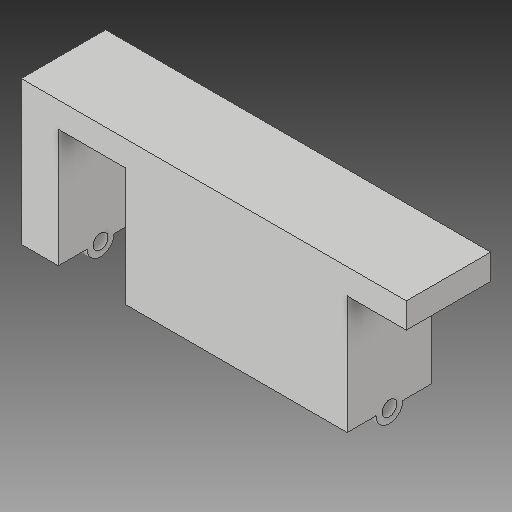
# Autodesk Inventor part: Arm_Base
Saved by Autodesk Inventor 2017 (Build 210142000, 142)
## iProperties
Created: 2016-12-31
Part Number: Arm_Base
Material: Generic
Document SubType Name: Modeling
Designer: Samanth
Density: 1 g/cm^3
Appearance: Default
Author: Samanth
Autodesk Inventor part; units mm, degrees
ref_plane "YZ Plane" through (0, 0, 0) normal (1, 0, 0) x (0, 1, 0)
ref_plane "XZ Plane" through (0, 0, 0) normal (0, 1, 0) x (-1, 0, 0)
ref_plane "XY Plane" through (0, 0, 0) normal (0, 0, 1) x (1, 0, 0)
sketch "Sketch1" plane through (0, 0, 0) normal (0, 0, 1) x (1, 0, 0)
  line L0 (0, 0) -> (55, 0)
  line L1 (0, 0) -> (-76, 0)
  line L2 (-116, 0) -> (-138, 0)
  line L3 (-138, 0) -> (-138, 70)
  line L4 (-138, 70) -> (-138, 85)
  line L5 (-138, 85) -> (-116, 85)
  line L6 (-116, 0) -> (-116, 70)
  line L7 (-116, 70) -> (-76, 70)
  line L8 (-76, 70) -> (-76, 0)
  line L9 (90, 70) -> (90, 85)
  line L10 (90, 85) -> (-116, 85)
  line L11 (55, 0) -> (55, 70)
  line L12 (55, 70) -> (90, 70)
  line L13 (55, 0) -> (-76, 0)
  line L14 (-116, 0) -> (-117.6, 0)
  line L15 (-117.6, 0) -> (-117.6, 71.4164)
  line L16 (-117.6, 71.4164) -> (-74.4045, 71.4164)
  line L17 (-74.4045, 71.4164) -> (-74.4045, 0)
  line L18 (-138, 0) -> (-152.8138, 0)
  line L19 (-152.8138, 0) -> (-152.8138, 85)
  line L20 (-152.8138, 85) -> (-138, 85)
  dimension "d20" = 1.6
  constraints: 42 end point, 10 perpendicular, 4 point on line, 4 vertical, 2 horizontal, 1 collinear
  measures "d20" distance of L2.start L14.end
extrude "Extrusion1" add sketch "Sketch1" along normal blind 50 contours L1 L17 L16 L15 L2 L3 L4 L5 L10 L9 L12 L11 L0 | L1 L8 L7 L6 L2 L15 L16 L17
sketch "Sketch2" plane through (0, 0, 0) normal (1, 0, 0) x (0, 1, 0)
  point P0 (0, 0)
sketch "Sketch3" plane through (-76, 0, 0) normal (0, -1, 0) x (1, 0, 0)
  line L0 (131, 0) -> (131, 50) projected
  line L1 (131, 25) -> (76, 25)
  circle A0 centre (76, 25) radius 2.5
  point P0 (76, 0)
  dimension "d9" = 5
  constraints: 2 end point, 1 centre point, 1 coincident, 1 horizontal, 1 midpoint
  measures "d9" diameter of A0
extrude "Extrusion2" cut sketch "Sketch3" against normal blind 50
sketch "Sketch4" plane through (55, 0, 0) normal (1, 0, 0) x (0, 0, -1)
  line L0 (0, 0) -> (-50, 0) projected
  circle A0 centre (-25, 0) radius 4.4
  dimension "d12" = 8.8
  constraints: 1 centre point, 1 midpoint
  measures "d12" diameter of A0
extrude "Extrusion3" cut sketch "Sketch4" against normal blind 238.5
sketch "Sketch5" plane through (55, 0, 0) normal (1, 0, 0) x (0, 0, -1)
  arc A0 (-20.6, 0) -> (-29.4, 0) centre (-25, 0) ccw projected
  circle A1 centre (-25, 0) radius 8
  circle A2 centre (-25, 0) radius 4.4
  point P0 (0, 0)
  dimension "d15" = 16
  constraints: 2 centre point, 2 coincident
  measures "d15" diameter of A1
extrude "Extrusion4" add sketch "Sketch5" against normal up to surface (193 mm away)
sketch "Sketch6" plane through (0, 0, 50) normal (0, 0, 1) x (1, 0, 0)
  line L0 (-116, 0) -> (-116, 70) projected
  line L1 (-116, 13.3517) -> (-76, 13.3517)
  line L2 (-76, 13.3517) -> (-76, -16.9742)
  line L3 (-76, -16.9742) -> (-116, -16.9742)
  line L4 (-116, -16.9742) -> (-116, 13.3517)
  point P0 (0, 0)
  constraints: 8 end point, 2 parallel, 1 horizontal, 1 perpendicular, 1 point on line
extrude "Extrusion5" cut sketch "Sketch6" against normal blind 238.5
body "Solid1"
